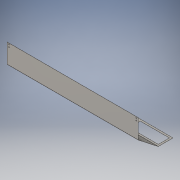
# Autodesk Inventor part: MC Part1
Saved by Autodesk Inventor 2016 (Build 200138000, 138)
## iProperties
Created: 2017-10-17
Part Number: MC Part1
Material: Steel, Mild
Document SubType Name: Sheet Metal
Designer: m207653
Density: 7.85 g/cm^3
Sheet Metal Rule: ms Steel
Appearance: Semi-Polished
Flat Pattern Width: 76.9396 cm
Flat Pattern Length: 169.5 cm
Flat Pattern Area: 13041.3 cm^2
Sheet Metal Width: 769.396 mm
Sheet Metal Length: 1695.000 mm
Sheet Metal Area: 1304125.843 mm^2
Author: m207653
Autodesk Inventor part; units mm, degrees
ref_plane "YZ Plane" through (0, 0, 0) normal (1, 0, 0) x (0, 1, 0)
ref_plane "XZ Plane" through (0, 0, 0) normal (0, 1, 0) x (-1, 0, 0)
ref_plane "XY Plane" through (0, 0, 0) normal (0, 0, 1) x (1, 0, 0)
sketch "Sketch1" plane through (0, 0, 0) normal (0, 0, 1) x (1, 0, 0)
  line L0 (0, 0) -> (0, 190)
  line L1 (0, 190) -> (1695, 190)
  line L2 (1695, 190) -> (1695, 0)
  line L3 (1695, 0) -> (0, 0)
  dimension "d0" = 190
  dimension "d1" = 1695
  measures "d0" distance of L0.start L0.end
  measures "d1" distance of L0.end L1.end
extrude "Plate1" add sketch "Sketch1" along normal blind 1.6
sketch "Sketch2" plane through (0, -0.9851, 1.9392) normal (0, -0.6156615, -0.7880108) x (1, 0, 0)
  line L0 (1695, 0) -> (0, 0)
  line L1 (0, 0) -> (0, -328.8982)
  line L2 (0, -328.8982) -> (1695, -328.8982)
  line L3 (1695, -328.8982) -> (1695, 0)
  constraints: 6 end point, 1 horizontal, 1 perpendicular, 1 vertical
edge flange "Flange1" height 330 angle 38 thickness 1.6 bend radius 1.6 thickness toward (0, -0.6156615, -0.7880108) relief straight relief width 1.6 relief depth 0.8 edges at (847.5, 0, 0) wall of the first edge with corners at (1695, -0.9851, 1.9392) (0, -0.9851, 1.9392) (0, -260.1603, 204.4291) (1695, -260.1603, 204.4291)
bend "Bend1"
corner "Corner1"
sketch "Sketch3" plane through (0, -259.5454, 203.1683) normal (0, -1, 0) x (1, 0, 0)
  line L0 (1695, 0) -> (0, 0)
  line L1 (0, 0) -> (0, -250)
  line L2 (0, -250) -> (1695, -250)
  line L3 (1695, -250) -> (1695, 0)
  constraints: 6 end point, 1 horizontal, 1 perpendicular, 1 vertical
edge flange "Flange2" height 250 angle 52 thickness 1.6 bend radius 1.6 thickness toward (0, -1, 0) relief straight relief width 1.6 relief depth 0.8 edges at (847.5, -261.1454, 203.1683) wall of the first edge with corners at (1695, -259.5454, 203.1683) (0, -259.5454, 203.1683) (0, -259.5454, 453.1683) (1695, -259.5454, 453.1683)
bend "Bend2"
corner "Corner2"
sketch "Sketch4" plane through (0, -259.5454, 453.1683) normal (0, 1, 0) x (1, 0, 0)
  line L0 (1695, 248.4393) -> (1695, 0) projected
  line L1 (1695, 60) -> (0, 60)
  line L2 (0, 248.4393) -> (0, 0) projected
  line L3 (1695, 0) -> (0, 0) projected
  circle A0 centre (1670, 15) radius 6
  circle A1 centre (1670, 45) radius 6
  circle A2 centre (25, 15) radius 6
  circle A3 centre (25, 45) radius 6
  point P0 (0, 453.1683)
  dimension "d23" = 60
  dimension "d24" = 12
  dimension "d25" = 12
  dimension "d26" = 25
  dimension "d27" = 25
  dimension "d28" = 15
  dimension "d29" = 15
  dimension "d30" = 12
  dimension "d31" = 12
  dimension "d32" = 25
  dimension "d33" = 25
  dimension "d41" = 15
  dimension "d42" = 15
  constraints: 4 centre point, 2 end point, 2 point on line, 1 horizontal
  measures "d23" distance between parallel lines of L3 L1
  measures "d24" diameter of A0
  measures "d25" diameter of A1
  measures "d26" distance from line of L0 A0.centre
  measures "d27" distance from line of L0 A1.centre
  measures "d28" distance from line of L3 A0.centre
  measures "d29" distance from line of L1 A1.centre
  measures "d30" diameter of A2
  measures "d31" diameter of A3
  measures "d32" distance from line of L2 A2.centre
  measures "d33" distance from line of L2 A3.centre
  measures "d41" distance from line of L3 A2.centre
  measures "d42" distance from line of L1 A3.centre
hole "Hole1" at (1670, -259.5454, 438.1683) at (1670, -259.5454, 408.1683) at (25, -259.5454, 438.1683) at (25, -259.5454, 408.1683) direction (0, -1, 0) diameter 12 end through all
sketch "Sketch5" plane through (0, 0, 1.6) normal (0, 0, 1) x (1, 0, 0)
  line L0 (1695, 190) -> (1695, 0) projected
  line L1 (0, 190) -> (1695, 190) projected
  line L2 (1695, 0) -> (1273, 0)
  line L3 (1273, 0) -> (1273, 190)
  line L4 (1273, 190) -> (1695, 190)
  line L5 (1695, 190) -> (1695, 0)
  line L6 (1672, 23) -> (1296, 23)
  line L7 (1296, 23) -> (1296, 167)
  line L8 (1296, 167) -> (1672, 167)
  line L9 (1672, 167) -> (1672, 23)
  point P0 (0, 0)
  dimension "d43" = 422
  dimension "d44" = 23
  dimension "d45" = 23
  dimension "d46" = 23
  dimension "d47" = 23
  constraints: 16 end point, 4 parallel, 2 horizontal, 2 perpendicular, 1 point on line
  measures "d43" distance of L3.end L4.end
  measures "d44" distance between parallel lines of L2 L6
  measures "d45" distance between parallel lines of L3 L7
  measures "d46" distance between parallel lines of L0 L9
  measures "d47" distance between parallel lines of L1 L8
extrude "Cut1" cut sketch "Sketch5" against normal blind 1.6 contours L6 L7 L8 L9
equation "\"d39\" = Thickness"
equation "\"d48\" = Thickness"
equation "\"d3\" = BendReliefWidth"
equation "\"d4\" = BendReliefDepth"
equation "\"d5\" = MinimumRemnant"
equation "\"d6\" = BendRadius"
equation "\"d9\" = BendRadius"
equation "\"d10\" = CornerReliefSize"
equation "\"d11\" = GapSize"
equation "\"d12\" = JacobiRadiusSize"
equation "\"d13\" = BendReliefWidth"
equation "\"d14\" = BendReliefDepth"
equation "\"d15\" = MinimumRemnant"
equation "\"d16\" = BendRadius"
equation "\"d19\" = BendRadius"
equation "\"d20\" = CornerReliefSize"
equation "\"d21\" = GapSize"
equation "\"d22\" = JacobiRadiusSize"
equation "\"BendRadius\" = Thickness"
equation "\"BendReliefWidth\" = Thickness"
equation "\"BendReliefDepth\" = 0.5 * Thickness"
equation "\"CornerReliefSize\" = 4 * Thickness"
equation "\"MinimumRemnant\" = 2 * Thickness"
equation "\"TransitionRadius\" = BendRadius"
equation "\"JacobiRadiusSize\" = BendRadius"
equation "\"GapSize\" = Thickness"
equation "\"d2\" = BendRadius"
equation "\"Thickness\" = 1.6"
body "Solid1"
